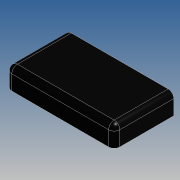
# Autodesk Inventor part: P304CouvercleBatterie
Saved by Autodesk Inventor 2015 SP1 (Build 190203100, 203)
## iProperties
Created: 2017-01-31
Part Number: P304CouvercleBatterie
Material: ABS Plastic
Document SubType Name: Modeling
Designer: serge.amoos
Density: 1.06 g/cm^3
Appearance: Smooth - Black
Author: serge.amoos
Autodesk Inventor part; units mm, degrees
ref_plane "YZ Plane" through (0, 0, 0) normal (1, 0, 0) x (0, 1, 0)
ref_plane "XZ Plane" through (0, 0, 0) normal (0, 1, 0) x (-1, 0, 0)
ref_plane "XY Plane" through (0, 0, 0) normal (0, 0, 1) x (1, 0, 0)
sketch "Sketch1" plane through (0, 0, 0) normal (0, 0, 1) x (1, 0, 0)
  line L0 (-34.8, 0) -> (5.8, 0) construction
  line L1 (0, -38.4) -> (0, 6.4) construction
  line L2 (0, 0) -> (-29, 0)
  line L3 (-29, 0) -> (-29, -32)
  line L4 (-29, -32) -> (0, -32)
  line L5 (0, -32) -> (0, 0)
  dimension "d0" = 29
  dimension "d1" = 32
  constraints: 8 end point, 2 parallel, 1 horizontal, 1 perpendicular
  measures "d0" distance of L3.end L4.end
  measures "d1" distance of L2.end L3.end
extrude "Extrusion1" add sketch "Sketch1" along normal blind 11
fillet "Fillet1" radius 3 1 edges at (-29, -32, 5.5)
fillet "Fillet2" radius 3 3 edges at (-28.1213, -31.1213, 11) (-29, -14.5, 11) (-13, -32, 11)
shell "Shell1" thickness 2 removed faces 3 at (-9.6667, -20.3333, 0) at (-18.3333, 0, 3.6667) at (0, -20.3333, 3.6667)
sketch "Sketch3" plane through (0, 0, 0) normal (0, 0, -1) x (-1, 0, 0)
  line L0 (27, 0) -> (27, -29) projected
  arc A0 (26, -30) -> (27, -29) centre (26, -29) ccw projected
  line L1 (26, -30) -> (0, -30) projected
  line L2 (28, 0) -> (28, -29)
  arc A1 (26, -31) -> (28, -29) centre (26, -29) ccw
  line L3 (26, -31) -> (0, -31)
  line L4 (27, 0) -> (28, 0)
  line L5 (0, -30) -> (0, -31)
  point P0 (0, 0)
  dimension "d19" = 1
  constraints: 8 end point, 2 point on circle, 1 centre point, 1 horizontal, 1 perpendicular, 2 other
  measures "d19" distance between parallel lines of L2 L0
extrude "Extrusion3" cut sketch "Sketch3" against normal blind 2
sketch "Sketch4" plane through (0, 0, 0) normal (0, 0, -1) x (-1, 0, 0)
  line L0 (0, -31) -> (26, -31) construction
  arc A0 (26, -31) -> (28, -29) centre (26, -29) ccw construction
  line L1 (28, -29) -> (28, 0) construction
  line L2 (28, 0) -> (29, 0) construction
  line L3 (29, 0) -> (29, -29) construction
  arc A1 (26, -32) -> (29, -29) centre (26, -29) ccw construction
  line L4 (26, -32) -> (0, -32) construction
  line L5 (0, -32) -> (0, -31) construction
  line L6 (28, 0) -> (27.6, 0)
  line L7 (27.6, 0) -> (27.6, -3)
  line L8 (27.6, -3) -> (28, -3)
  line L9 (28, -3) -> (28, 0)
  line L10 (28, -12) -> (27.8, -12)
  line L11 (27.8, -12) -> (27.8, -22)
  line L12 (27.8, -22) -> (28, -22)
  line L13 (28, -22) -> (28, -12)
  line L14 (0, -31) -> (5, -31)
  line L15 (5, -31) -> (5, -30.8)
  line L16 (5, -30.8) -> (0, -30.8)
  line L17 (0, -30.8) -> (0, -31)
  point P0 (0, 0)
  dimension "d22" = 5
  dimension "d23" = 0.2
  dimension "d24" = 0.2
  dimension "d25" = 10
  dimension "d26" = 10
  dimension "d27" = 3
  dimension "d28" = 0.4
  constraints: 24 end point, 6 parallel, 3 horizontal, 3 perpendicular, 1 point on line
  measures "d22" distance of L15.end L16.end
  measures "d23" distance of L14.end L15.end
  measures "d24" distance of L11.end L12.end
  measures "d25" distance of L10.end L11.end
  measures "d26" distance from line of L4 L11.end
  measures "d27" distance of L6.end L7.end
  measures "d28" distance between parallel lines of L1 L7
extrude "Extrusion4" add sketch "Sketch4" against normal blind 0.8
chamfer "Chamfer2" distance 0.4 angle 45 1 edges at (-27.6, -3, 0.4)
fillet "Fillet4" radius 0.2 3 edges at (-27.6, -1.3001, 0.8) (-27.8, -17, 0.8) (-2.5, -30.8, 0.8)
mirror "Mirror1" about plane through (0, -32, 0) normal (1, 0, 0)
body "Solid1"
